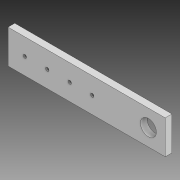
# Autodesk Inventor part: backplate
Saved by Autodesk Inventor 2020 (Build 240168000, 168)
## iProperties
Created: 2020-11-25
Part Number: backplate
Material: Generic
Document SubType Name: Modeling
Designer: DDeGo
Density: 1 g/cm^3
Appearance: Default
Author: DDeGo
Autodesk Inventor part; units mm, degrees
ref_plane "YZ Plane" through (0, 0, 0) normal (1, 0, 0) x (0, 1, 0)
ref_plane "XZ Plane" through (0, 0, 0) normal (0, 1, 0) x (-1, 0, 0)
ref_plane "XY Plane" through (0, 0, 0) normal (0, 0, 1) x (1, 0, 0)
sketch "Sketch1" plane through (0, 0, 0) normal (0, 0, 1) x (1, 0, 0)
  line L0 (-70, -15) -> (70, -15)
  line L1 (70, -15) -> (70, 15)
  line L2 (70, 15) -> (-70, 15)
  line L3 (-70, 15) -> (-70, -15)
  line L4 (-70, -15) -> (70, 15) construction
  line L5 (70, -15) -> (-70, 15) construction
  line L6 (0, 0) -> (55, 0) construction
  circle A0 centre (55, 0) radius 7.1238
  line L7 (0, 0) -> (5, 0) construction
  circle A1 centre (5, 0) radius 1.5
  circle A2 centre (-15, 0) radius 1.5
  circle A3 centre (-35, 0) radius 1.5
  circle A4 centre (-55, 0) radius 1.5
  dimension "d1" = 30
  dimension "d2" = 140
  dimension "d3" = 15
  dimension "d4" = 50
  dimension "d7" = 20
  dimension "d12" = 3
  constraints: 16 end point, 5 centre point, 3 horizontal, 2 coincident, 2 midpoint, 2 parallel, 1 perpendicular, 1 point on line, 6 other
  measures "d1" distance of L0.end L1.end
  measures "d2" distance of L0.start L0.end
  measures "d3" distance from line of L1 L6.end
  measures "d4" distance of L6.end L7.end
  measures "d7" distance of A1.centre A2.centre
  measures "d12" diameter of A1
extrude "Extrusion1" add sketch "Sketch1" along normal blind 6
body "Solid1"
